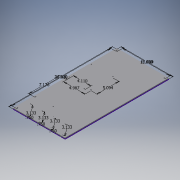
# Autodesk Inventor part: eboardbaseplate
Saved by Autodesk Inventor 2016 (Build 200138000, 138)
## iProperties
Created: 2016-01-21
Part Number: eboardbaseplate
Material: Generic
Document SubType Name: Modeling
Designer: Administrator
Density: 1 g/cm^3
Appearance: Default
Author: Administrator
Autodesk Inventor part; units mm, degrees
ref_plane "YZ Plane" through (0, 0, 0) normal (1, 0, 0) x (0, 1, 0)
ref_plane "XZ Plane" through (0, 0, 0) normal (0, 1, 0) x (-1, 0, 0)
ref_plane "XY Plane" through (0, 0, 0) normal (0, 0, 1) x (1, 0, 0)
sketch "Sketch1" plane through (0, 0, 0) normal (0, 1, 0) x (-1, 0, 0)
  line L0 (-139.7, 292.1) -> (139.7, 292.1)
  line L1 (139.7, 292.1) -> (139.7, -292.1)
  line L2 (139.7, -292.1) -> (-139.7, -292.1)
  line L3 (-139.7, -292.1) -> (-139.7, 292.1)
  line L4 (-139.7, 292.1) -> (139.7, -292.1) construction
  line L5 (139.7, 292.1) -> (-139.7, -292.1) construction
  line L6 (-152.4, 304.8) -> (152.4, 304.8)
  line L7 (152.4, 304.8) -> (152.4, -304.8)
  line L8 (152.4, -304.8) -> (-152.4, -304.8)
  line L9 (-152.4, -304.8) -> (-152.4, 304.8)
  line L10 (-152.4, 304.8) -> (152.4, -304.8) construction
  line L11 (152.4, 304.8) -> (-152.4, -304.8) construction
  line L12 (40.5945, 180.2806) -> (144.9885, 180.2806)
  line L13 (144.9885, 180.2806) -> (144.9885, -1.9898)
  line L14 (144.9885, -1.9898) -> (40.5945, -1.9898)
  line L15 (40.5945, -1.9898) -> (40.5945, 180.2806)
  line L16 (40.5945, 180.2806) -> (144.9885, -1.9898) construction
  line L17 (144.9885, 180.2806) -> (40.5945, -1.9898) construction
  line L18 (144.2829, -147.4078) -> (17.6131, -147.4078)
  line L19 (17.6131, -147.4078) -> (17.6131, -18.0202)
  line L20 (17.6131, -18.0202) -> (144.2829, -18.0202)
  line L21 (144.2829, -18.0202) -> (144.2829, -147.4078)
  line L22 (144.2829, -147.4078) -> (17.6131, -18.0202) construction
  line L23 (17.6131, -147.4078) -> (144.2829, -18.0202) construction
  line L24 (122.3815, 294.9298) -> (73.9219, 294.9298)
  line L25 (73.9219, 294.9298) -> (73.9219, 231.8081)
  line L26 (73.9219, 231.8081) -> (122.3815, 231.8081)
  line L27 (122.3815, 231.8081) -> (122.3815, 294.9298)
  line L28 (122.3815, 294.9298) -> (73.9219, 231.8081) construction
  line L29 (54.8719, 294.9298) -> (6.4122, 294.9298)
  line L30 (6.4122, 294.9298) -> (6.4122, 231.8081)
  line L31 (6.4122, 231.8081) -> (54.8719, 231.8081)
  line L32 (54.8719, 231.8081) -> (54.8719, 294.9298)
  line L33 (-12.6378, 294.9298) -> (-61.0974, 294.9298)
  line L34 (-61.0974, 294.9298) -> (-61.0974, 231.8081)
  line L35 (-61.0974, 231.8081) -> (-12.6378, 231.8081)
  line L36 (-12.6378, 231.8081) -> (-12.6378, 294.9298)
  line L37 (-80.1474, 294.9298) -> (-128.607, 294.9298)
  line L38 (-128.607, 294.9298) -> (-128.607, 231.8081)
  line L39 (-128.607, 231.8081) -> (-80.1474, 231.8081)
  line L40 (-80.1474, 231.8081) -> (-80.1474, 294.9298)
  line L41 (73.9219, 294.9298) -> (122.3815, 231.8081)
  line L42 (6.4122, 294.9298) -> (54.8719, 231.8081)
  line L43 (-61.0974, 294.9298) -> (-12.6378, 231.8081)
  line L44 (-128.607, 294.9298) -> (-80.1474, 231.8081)
  point P0 (0, 0)
  point P1 (0, 0)
  point P2 (0, 0)
  point P3 (92.7915, 89.1454)
  point P4 (92.7915, 89.1454)
  point P5 (80.948, -82.714)
  point P6 (80.948, -82.714)
  point P7 (98.1517, 263.3689)
  dimension "d71" = 279.4
  dimension "d72" = 584.2
  dimension "d73" = 304.8
  dimension "d74" = 609.6
  dimension "d84" = 104.394
  dimension "d85" = 182.2704
  dimension "d86" = 126.6698
  dimension "d87" = 129.3876
  dimension "d102" = 19.05
  dimension "d103" = 19.05
  dimension "d104" = 19.05
  dimension "d112" = 79.5782
  dimension "d113" = 79.5782
  dimension "d114" = 79.5782
  dimension "d115" = 79.5782
  constraints: 90 end point, 20 coincident, 16 parallel, 13 midpoint, 8 horizontal, 8 perpendicular, 2 point on line, 3 other
  measures "d71" distance of L1.end L2.end
  measures "d72" distance of L0.end L1.end
  measures "d73" distance of L7.end L8.end
  measures "d74" distance of L6.end L7.end
  measures "d84" distance of L13.end L14.end
  measures "d85" distance of L12.end L13.end
  measures "d86" distance of L19.end L20.end
  measures "d87" distance of L18.end L19.end
  measures "d102" distance of L29.start L24.end
  measures "d103" distance of L33.start L29.end
  measures "d104" distance of L37.start L33.end
  measures "d112" distance of L41.start L41.end
  measures "d113" distance of L31.end L29.end
  measures "d114" distance of L35.end L33.end
  measures "d115" distance of L39.end L37.end
extrude "Extrusion6" add sketch "Sketch1" along normal blind 6.35 contours L0 L38 L39 L40 L34 L35 L36 L30 L31 L32 L25 L26 L27 L1 L12 L15 L14 L20 L19 L18 L2 L3 | L38 L44 L0 | L0 L44 L39 L38 | L44 L37 L40 L0 | L0 L40 L44 | L18 L19 L20 L1 | L1 L20 L21 L18 | L34 L43 L0 | L0 L43 L35 L34 | L43 L33 L36 L0 | L0 L36 L43 | L14 L15 L12 L1 | L1 L12 L13 L14 | L30 L42 L0 | L0 L42 L31 L30 | L42 L29 L32 L0 | L0 L32 L42 | L27 L41 L0 | L0 L41 L24 L27 | L41 L26 L25 L0 | L0 L25 L41 | L6 L7 L8 L9
hole "Hole6" at (139.7, 0, 292.1) at (-139.7, 0, 292.1) at (-139.7, 0, -292.1) at (139.7, 0, -292.1) at (-17.6131, 0, -18.0202) at (-17.6131, 0, -147.4078) at (-144.2829, 0, -147.4078) at (-144.2829, 0, -18.0202) at (-144.9885, 0, 180.2806) at (-40.5945, 0, 180.2806) at (-40.5945, 0, -1.9898) at (-144.9885, 0, -1.9898) direction (0, 1, 0) diameter 6.35 end through all
hole "Hole7" at (-122.3815, 0, 231.8081) at (-73.9219, 0, 294.9298) at (-54.8719, 0, 231.8081) at (-6.4122, 0, 294.9298) at (12.6378, 0, 231.8081) at (61.0974, 0, 294.9298) at (80.1474, 0, 231.8081) at (128.607, 0, 294.9298) direction (0, 1, 0) diameter 3.81 end through all
body "Solid6"
